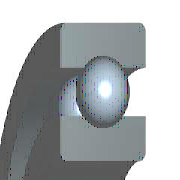
# Autodesk Inventor part: DIN 625 SKF - SKF 6205
Saved by Autodesk Inventor 2023 (Build 270158000, 158)
## iProperties
Created: 2022-02-04
Part Number: DIN 625 SKF - SKF 6205
Material: Сталь, мягкая
Description: Подшипники шариковые однорядные SKF
Document SubType Name: Modeling
Standard: DIN 625 SKF
Designer: Josh
Standards Organization: DIN
Language: ru-RU
Size Designation: SKF 6205
Categories: <MemberInstance><Categories><Category DisplayName="Детали вала" InternalName="7f7aeb1f-a693-4053-b835-cee3144e0d98" Mnemonic="SHFT"><Category DisplayName="Подшипники" InternalName="242d30a3-7172-44e6-a363-b0a3d8f1b556" Mnemonic="BRNG"><CategoryParameter DisplayName="Ширина" InternalName="25fc5f6e-338b-4801-b5ed-8959743e396e" Mnemonic="wdth"/><CategoryParameter DisplayName="Обозначение размера" InternalName="2c4e891a-c8f4-49ed-a5c1-5131476c6feb" Mnemonic="sizedes"/><CategoryParameter DisplayName="Номинальная динамическая нагрузка" InternalName="440972dd-7009-4861-bd45-69ffbb461423" Mnemonic="bdynlrat"/><CategoryParameter DisplayName="Диаметр вала" InternalName="91302473-2833-4451-a660-c5d4a8d6a031" Mnemonic="shaftdia"/><CategoryParameter DisplayName="Угол касания" InternalName="aa21a452-7974-4a55-b5cf-1c2972de2aea" Mnemonic="TouchAngle"/><CategoryParameter DisplayName="Наружный диаметр" InternalName="d441686c-04bd-4681-b674-94fbc173ec23" Mnemonic="outdia"/><Category DisplayName="Подшипники шариковые" InternalName="9b553946-0899-4a5e-a403-c1d9295e77c1" Mnemonic="BALLBEAR"><CategoryParameter DisplayName="Коэффициент радиальной динамической нагрузки при Fa/Fr  &lt;= e" InternalName="051e59b3-bd55-4dad-8b07-38b5cb912881" Mnemonic="raddynfc1"/><CategoryParameter DisplayName="Номинальная статическая нагрузка" InternalName="0f13fbbf-c511-4d43-b4c7-197b47424baf" Mnemonic="bstatlrat"/><CategoryParameter DisplayName="Ресурс" InternalName="3029e2ef-9460-4be8-bdfd-dfe61437473d" Mnemonic="lifeexp"/><CategoryParameter DisplayName="Коэффициент трения" InternalName="3086b0f2-3d69-46ff-8a75-fe12e395bb47" Mnemonic="fricfct"/><CategoryParameter DisplayName="Мин. диаметр вала" InternalName="4a5be9bc-ad86-4bf2-8167-102dad5d3e27" Mnemonic="minshaftdia"/><CategoryParameter DisplayName="Коэффициент осевой динамической нагрузки при Fa/Fr &gt; e" InternalName="4b6ff741-5956-4a40-80f5-34eb9259f88c" Mnemonic="axdynfc2"/><CategoryParameter DisplayName="Ограничивающая скорость смазка" InternalName="5237843b-2c8d-46d3-8227-f3e9dd85a12e" Mnemonic="lubgrsp"/><CategoryParameter DisplayName="Ограничивающее скорость масло" InternalName="60628548-8907-44dc-8e09-603d72f5766f" Mnemonic="oilspd"/><CategoryParameter DisplayName="Коэффициент осевой статической нагрузки" InternalName="74dbf5e2-8362-409a-802f-3c2235668d99" Mnemonic="axdynfc0"/><CategoryParameter DisplayName="Масса" InternalName="7b80f85c-da81-4dea-b8db-d7c689da91b2" Mnemonic="mass"/><CategoryParameter DisplayName="Радиус" InternalName="83352640-dfae-4cba-bc9f-11ecbfb0001c" Mnemonic="rad"/><CategoryParameter DisplayName="Коэффициент радиальной статической нагрузки" InternalName="83ce084d-c51e-4598-a871-e8e1e34b26ee" Mnemonic="raddynfc0"/><CategoryParameter DisplayName="Коэффициент осевой динамической нагрузки при Fa/Fr &lt;= e" InternalName="ae45a7db-08df-4411-99a8-2f035015bff9" Mnemonic="axdynfc1"/><CategoryParameter DisplayName="Макс. диаметр отсека втулки" InternalName="b5cf89e0-ca87-439c-b08c-a25e2999ab06" Mnemonic="maxhubdia"/><CategoryParameter DisplayName="Граничное значение для определения коэффициента" InternalName="be0ce6fc-cad4-4218-b484-c34dd2571812" Mnemonic="limvalfac"/><CategoryParameter DisplayName="Коэффициент радиальной динамической нагрузки при Fa/Fr &gt; e" InternalName="e513bdb7-139f-4b3c-af32-49e0ba1226b9" Mnemonic="raddynfc2"/><CategoryParameter DisplayName="Макс. радиус отсека скругления" InternalName="f6ce6695-cf2c-4ec9-8d20-66671e0e35a4" Mnemonic="maxstprad"/><Category DisplayName="Подшипники шариковые с глубоким желобом" InternalName="6f040212-0f73-4fa8-b5e4-17d6525fdc38" Mnemonic="BBDGBB"/></Category></Category></Category><Category DisplayName="ТипДанных" InternalName="23b78d0f-2648-40c6-8793-ca6db495c9e8" Mnemonic="DATATYPE"><CategoryParameter DisplayName="ОтображаемоеИмя" InternalName="05415f3d-3907-474b-a020-eb9d644f4cf3" Mnemonic="DISPLAYNAME"/><CategoryParameter DisplayName="Стандарт" InternalName="0c0a119c-1e12-4c84-803f-101930972f5e" Mnemonic="STANDARD"/><CategoryParameter DisplayName="Наименование" InternalName="13903e3d-64b1-4950-80da-f627842ea37f" Mnemonic="DESCRIPTION"/><CategoryParameter DisplayName="Обозначение" InternalName="2675968c-4ce5-49e0-a4f5-552d29089031" Mnemonic="DESIGNATION"/><CategoryParameter DisplayName="Строка по умолчанию" InternalName="2af9ec52-faaa-4026-b378-f9fa4afca842" Mnemonic="DEFAULTROW"/><CategoryParameter DisplayName="Имя папки" InternalName="3f06958e-8713-4116-9be7-ed6184ecc97b" Mnemonic="FOLDERNAME"/><CategoryParameter DisplayName="Указатель редакций" InternalName="45a75005-10b1-4dfc-8d6d-dfe629f0b93c" Mnemonic="REVISIONGUID"/><CategoryParameter DisplayName="ИмяФайла" InternalName="8b46a4cc-9585-4fed-90c3-899f57e09a73" Mnemonic="FILENAME"/><CategoryParameter DisplayName="ОргСтанд" InternalName="8f5914e1-4693-403f-8ab5-d37768198c9d" Mnemonic="STDSORG"/><CategoryParameter DisplayName="Версия семейства" InternalName="914462f6-6e19-4b14-ba84-155b9680b1d0" Mnemonic="FAMILYREVISION"/><CategoryParameter DisplayName="Редакция стандарта" InternalName="91d5a463-65c2-4fde-b823-3b7fea5e8e17" Mnemonic="STANDARDREVISION"/><CategoryParameter DisplayName="редакция элемента" InternalName="a65d44b9-392f-4f4f-857b-e4b3d54996fe" Mnemonic="MEMBERREVISION"/><CategoryParameter DisplayName="ФорматКлипа" InternalName="bc51e27b-3422-4e78-93ef-cec197ddf230" Mnemonic="CLIPFORMAT"/><CategoryParameter DisplayName="Изготовитель" InternalName="cd6c7a72-a28a-4e50-99a9-2c7f4e13e5ad" Mnemonic="MANUFACTURER"/><CategoryParameter DisplayName="ВнутреннееИмя" InternalName="cf1d0246-76d9-4b4a-8305-fa0409afb5c1" Mnemonic="INTERNALNAME"/><CategoryParameter DisplayName="Метрическая" InternalName="e2385c5b-1ea4-4823-96a8-8de651266ec3" Mnemonic="ISMETRIC"/><Category DisplayName="Деталь" InternalName="c0e0b642-3bcb-4cc8-9e80-f96d35c4afa4" Mnemonic="PART"><CategoryParameter DisplayName="Номер детали" InternalName="016b6077-bfbe-49bd-92c9-d8d59c39c941" Mnemonic="PARTNUMBER"/><CategoryParameter DisplayName="Инвентарный номер" InternalName="4dba7c1c-e26c-444e-836c-b08b433409a8" Mnemonic="STOCKNUMBER"/><CategoryParameter DisplayName="Ключ материала" InternalName="5c9a8adb-dd2b-4535-b97f-0a94a95fe41f" Mnemonic="MATERIALKEY"/><CategoryParameter DisplayName="Материал" InternalName="818a152a-d3c3-49ca-80ee-df7d91421b8e" Mnemonic="MATERIAL"/></Category></Category><Category DisplayName="Схема предыдущей версии DA" InternalName="924fff40-ddd0-4eff-ad42-30e3774ef79e" Mnemonic="LEGACYMAPDA"><CategoryParameter DisplayName="DACookie" InternalName="316934ee-8fe1-4c7a-9c36-f2d79e1add1a" Mnemonic="DACOOKIE"/></Category></Categories><FamilyTemplate Id="N024630"><FamilyTemplateParameters><FamilyTemplateParameter ObjectType="kUserParameterObject" ValueType="xs:double" Id="1" ObjectReferenceKey="Diam"/><FamilyTemplateParameter ObjectType="kUserParameterObject" ValueType="xs:integer" Id="2" ObjectReferenceKey="DD"/><FamilyTemplateParameter ObjectType="kUserParameterObject" ValueType="xs:double" Id="3" ObjectReferenceKey="B"/><FamilyTemplateParameter ObjectType="kUserParameterObject" ValueType="xs:double" Id="4" ObjectReferenceKey="r"/><FamilyTemplateParameter ObjectType="kPropertyObject" ValueType="xs:string" Id="100" ObjectReferenceKey="{32853F0F-3444-11d1-9E93-0060B03C1CA6}" SubObjectId="52"/><FamilyTemplateParameter ObjectType="kPropertyObject" ValueType="xs:string" Id="105" ObjectReferenceKey="{32853F0F-3444-11d1-9E93-0060B03C1CA6}" SubObjectId="5"/><FamilyTemplateParameter ObjectType="kPartComponentDefinitionObject" ValueType="xs:string" Id="110" SubObjectId="Material"/></FamilyTemplateParameters></FamilyTemplate><CategoryParameterMap><ParamToTemplateMap><ParamToTemplate CategoryParameter="//CategoryParameter[@InternalName='05415f3d-3907-474b-a020-eb9d644f4cf3']" ConstantValue="DIN 625 SKF"/><ParamToTemplate CategoryParameter="//CategoryParameter[@InternalName='cf1d0246-76d9-4b4a-8305-fa0409afb5c1']" ConstantValue="3507F009-3A51-47D4-853B-61FE72BC2791"/><ParamToTemplate CategoryParameter="//CategoryParameter[@InternalName='3f06958e-8713-4116-9be7-ed6184ecc97b']" ConstantValue="DIN BEARING(1)"/><ParamToTemplate CategoryParameter="//CategoryParameter[@InternalName='914462f6-6e19-4b14-ba84-155b9680b1d0']" ConstantValue="10"/><ParamToTemplate CategoryParameter="//CategoryParameter[@InternalName='bc51e27b-3422-4e78-93ef-cec197ddf230']" ConstantValue="CF_INVENTOR.STDPARTS"/><ParamToTemplate CategoryParameter="//CategoryParameter[@InternalName='e2385c5b-1ea4-4823-96a8-8de651266ec3']" ConstantValue="true"/><ParamToTemplate CategoryParameter="//CategoryParameter[@InternalName='13903e3d-64b1-4950-80da-f627842ea37f']" ConstantValue="Single row ball bearings SKF"/><ParamToTemplate CategoryParameter="//CategoryParameter[@InternalName='8f5914e1-4693-403f-8ab5-d37768198c9d']" ConstantValue="DIN"/><ParamToTemplate CategoryParameter="//CategoryParameter[@InternalName='0c0a119c-1e12-4c84-803f-101930972f5e']" ConstantValue="DIN 625 SKF"/><ParamToTemplate CategoryParameter="//CategoryParameter[@InternalName='cd6c7a72-a28a-4e50-99a9-2c7f4e13e5ad']" TemplateParameter="104"/><ParamToTemplate CategoryParameter="//CategoryParameter[@InternalName='91d5a463-65c2-4fde-b823-3b7fea5e8e17']" TemplateParameter="103"/><ParamToTemplate CategoryParameter="//CategoryParameter[@InternalName='45a75005-10b1-4dfc-8d6d-dfe629f0b93c']" ConstantValue="9ce72b97-1790-415a-a26a-a47894b5e3a8"/><ParamToTemplate CategoryParameter="//CategoryParameter[@InternalName='2af9ec52-faaa-4026-b378-f9fa4afca842']" ConstantValue="10"/><ParamToTemplate CategoryParameter="//CategoryParameter[@InternalName='8b46a4cc-9585-4fed-90c3-899f57e09a73']" ConstantValue="DIN 625 SKF - SKF 6205"/><ParamToTemplate CategoryParameter="//CategoryParameter[@InternalName='a65d44b9-392f-4f4f-857b-e4b3d54996fe']" ConstantValue="6BFEAA8C-157C-49D5-9CE2-AD54B101689B"/><ParamToTemplate CategoryParameter="//CategoryParameter[@InternalName='0f13fbbf-c511-4d43-b4c7-197b47424baf']" ConstantValue="7800"/><ParamToTemplate CategoryParameter="//CategoryParameter[@InternalName='5237843b-2c8d-46d3-8227-f3e9dd85a12e']" ConstantValue="18000"/><ParamToTemplate CategoryParameter="//CategoryParameter[@InternalName='3086b0f2-3d69-46ff-8a75-fe12e395bb47']" ConstantValue="0,0015"/><ParamToTemplate CategoryParameter="//CategoryParameter[@InternalName='3029e2ef-9460-4be8-bdfd-dfe61437473d']" ConstantValue="3"/><ParamToTemplate CategoryParameter="//CategoryParameter[@InternalName='4a5be9bc-ad86-4bf2-8167-102dad5d3e27']" ConstantValue="30,6"/><ParamToTemplate CategoryParameter="//CategoryParameter[@InternalName='b5cf89e0-ca87-439c-b08c-a25e2999ab06']" ConstantValue="46,4"/><ParamToTemplate CategoryParameter="//CategoryParameter[@InternalName='f6ce6695-cf2c-4ec9-8d20-66671e0e35a4']" ConstantValue="1"/><ParamToTemplate CategoryParameter="//CategoryParameter[@InternalName='60628548-8907-44dc-8e09-603d72f5766f']" ConstantValue="28000"/><ParamToTemplate CategoryParameter="//CategoryParameter[@InternalName='83ce084d-c51e-4598-a871-e8e1e34b26ee']" ConstantValue="0,6"/><ParamToTemplate CategoryParameter="//CategoryParameter[@InternalName='74dbf5e2-8362-409a-802f-3c2235668d99']" ConstantValue="0,5"/><ParamToTemplate CategoryParameter="//CategoryParameter[@InternalName='051e59b3-bd55-4dad-8b07-38b5cb912881']" ConstantValue="1"/><ParamToTemplate CategoryParameter="//CategoryParameter[@InternalName='ae45a7db-08df-4411-99a8-2f035015bff9']" ConstantValue="0"/><ParamToTemplate CategoryParameter="//CategoryParameter[@InternalName='2c4e891a-c8f4-49ed-a5c1-5131476c6feb']" ConstantValue="6205"/><ParamToTemplate CategoryParameter="//CategoryParameter[@InternalName='316934ee-8fe1-4c7a-9c36-f2d79e1add1a']" ConstantValue="*DIN~N024630A~SKF 6205*"/><ParamToTemplate CategoryParameter="//CategoryParameter[@InternalName='25fc5f6e-338b-4801-b5ed-8959743e396e']" TemplateParameter="3"/><ParamToTemplate CategoryParameter="//CategoryParameter[@InternalName='d441686c-04bd-4681-b674-94fbc173ec23']" TemplateParameter="2"/><ParamToTemplate CategoryParameter="//CategoryParameter[@InternalName='2675968c-4ce5-49e0-a4f5-552d29089031']" TemplateParameter="100"/><ParamToTemplate CategoryParameter="//CategoryParameter[@InternalName='91302473-2833-4451-a660-c5d4a8d6a031']" TemplateParameter="1"/><ParamToTemplate CategoryParameter="//CategoryParameter[@InternalName='818a152a-d3c3-49ca-80ee-df7d91421b8e']" TemplateParameter="110"/><ParamToTemplate CategoryParameter="//CategoryParameter[@InternalName='016b6077-bfbe-49bd-92c9-d8d59c39c941']" TemplateParameter="105"/><ParamToTemplate CategoryParameter="//CategoryParameter[@InternalName='83352640-dfae-4cba-bc9f-11ecbfb0001c']" TemplateParameter="4"/></ParamToTemplateMap></CategoryParameterMap></MemberInstance>
Density: 7.85 g/cm^3
Appearance: С умеренной полировкой
IsCustomPart: 0
Author: Josh
Autodesk Inventor part; units mm, degrees
ref_plane "YZ Plane" through (0, 0, 0) normal (1, 0, 0) x (0, 1, 0)
sketch "Эскиз1" plane through (0, 0, 0) normal (0, 0, 1) x (1, 0, 0)
  point P0 (0, 0)
sketch "Эскиз2" plane through (0, 0, 0) normal (1, 0, 0) x (0, 1, 0)
  line L0 (12.5, 15) -> (26, 15)
  line L1 (12.5, 0) -> (12.5, 15)
  line L2 (26, 0) -> (12.5, 0)
  line L3 (26, 15) -> (26, 0)
  line L4 (0, 0) -> (0, 20) construction
  line L5 (0, 0) -> (0, 20)
  line L6 (-7.2, 0) -> (43.2, 0) projected
  dimension "d1" = 25
  dimension "d3" = 52
  dimension "d5" = 15
  constraints: 12 end point, 3 vertical, 2 horizontal, 1 collinear, 1 other
  measures "d1" diameter of L0.start L4
  measures "d3" diameter of L0.end L4
  measures "d5" distance of L1.start L0.start
revolve "Вращение1" add sketch "Эскиз2" angle 360 about axis through (0, 0, 0) along (0, 0, 1)
ref_plane "WorkPlane3" through (0, 0, 0) normal (0, 0, -1) x (-1, 0, 0)
sketch "Эскиз3" plane through (0, 0, 0) normal (1, 0, 0) x (0, 1, 0)
  arc A0 (21.68, 4.26) -> (21.68, 10.74) centre (19.25, 7.5) ccw
  line L0 (21.68, 15) -> (21.68, 10.74)
  line L1 (16.82, 15) -> (21.68, 15)
  line L2 (16.82, 10.74) -> (16.82, 15)
  arc A1 (16.82, 10.74) -> (16.82, 4.26) centre (19.25, 7.5) ccw
  line L3 (16.82, 0) -> (16.82, 4.26)
  line L4 (21.68, 0) -> (16.82, 0)
  line L5 (21.68, 4.26) -> (21.68, 0)
  line L6 (26, 0) -> (-26, 0) construction
  line L7 (26, 15) -> (-26, 15) construction
  line L8 (0, -42.2904) -> (0, 61.2904)
  line L9 (0, 82.0066) -> (0, -63.0066) projected
  dimension "d9" = 8.1
  dimension "d21" = 16.82
  dimension "d22" = 19.25
  dimension "d23" = 21.68
  constraints: 14 end point, 4 collinear, 4 point on circle, 4 vertical, 2 centre point, 2 concentric, 2 horizontal, 2 point on line
  measures "d9" diameter of A0
  measures "d21" distance between parallel lines of L8 L3
  measures "d22" distance from line of L8 A0.centre
  measures "d23" distance between parallel lines of L8 L5
revolve "Вращение2" cut sketch "Эскиз3" angle 360 about axis through (0, 0, -42.2904) along (0, 0, 1)
ref_plane "WorkPlane4" through (0, 0, 15) normal (0, 0, -1) x (-1, 0, 0)
sketch "Эскиз4" plane through (0, 0, 15) normal (0, 0, -1) x (-1, 0, 0)
  point P0 (0, 0)
sketch "Эскиз5" plane through (0, 0, 0) normal (1, 0, 0) x (0, 1, 0)
  arc A0 (19.25, 3.4499) -> (19.25, 11.55) centre (19.25, 7.5) ccw
  line L0 (19.25, 3.4499) -> (19.25, 11.55)
  line L1 (21.68, 0) -> (-21.68, 0) construction
  line L2 (19.25, 3.4499) -> (19.25, 11.55)
  arc A1 (21.68, 4.26) -> (21.68, 10.74) centre (19.25, 7.5) ccw projected
  dimension "d13" = 0
  dimension "d15" = 8.1001
  constraints: 4 end point, 2 point on circle, 1 centre point, 1 concentric, 1 vertical
  measures "d13" horizontal distance of A0.centre L0.start
  measures "d15" diameter of A0
revolve "Вращение3" add sketch "Эскиз5" angle 360 about axis through (0, 19.25, 3.4499) along (0, 0, 1)
pattern_circular "Круговой массив1" count 8 over 360 about axis through (0, 0, 7.5) along (0, 0, 1) of "Вращение3"
fillet "Сопряжение1" radius 1 4 edges at (0, -26, 15) (0, -26, 0) (0, -12.5, 15) (0, -12.5, 0)
equation "\"d17\" = msp_pocet"
equation "\"d20\" = r"
equation "\"d1\" = Diam"
equation "\"d3\" = DD"
equation "\"d5\" = msp_mdtd2"
equation "\"d9\" = msp_mdtd6"
equation "\"d21\" = 0.5 * msp_d1"
equation "\"d22\" = 0.5 * msp_ds"
equation "\"d23\" = 0.5 * msp_dd1"
equation "\"Diam\" = 25"
equation "\"DD\" = 52"
equation "\"B\" = 15"
equation "\"r\" = 1"
equation "\"msp_ds\" = 0.5 * Diam + 0.5 * DD"
equation "\"msp_d0\" = -0.3 * Diam + 0.3 * DD"
equation "\"msp_d1\" = msp_ds - 0.6 * msp_d0"
equation "\"msp_dd1\" = msp_ds + 0.6 * msp_d0"
equation "\"msp_pom\" = 1.5 * msp_ds"
equation "\"msp_mdtd2\" = B"
equation "\"msp_mdtd4\" = msp_ds"
equation "\"msp_mdtd6\" = msp_d0"
equation "\"msp_mdtd7\" = 0.5 * msp_mdtd2"
equation "\"msp_pocet\" = 7.52963"
body "Solid1"
